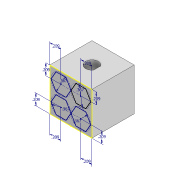
# Autodesk Inventor part: 615456 bevel gear lock A
Saved by Autodesk Inventor 2020 (Build 240168000, 168)
## iProperties
Created: 2019-11-11
Part Number: 615456 bevel gear lock A
Material: Generic
Document SubType Name: Modeling
Designer: ball
Density: 1 g/cm^3
Appearance: Default
Author: ball
Autodesk Inventor part; units mm, degrees
ref_plane "YZ Plane" through (0, 0, 0) normal (1, 0, 0) x (0, 1, 0)
ref_plane "XZ Plane" through (0, 0, 0) normal (0, 1, 0) x (-1, 0, 0)
ref_plane "XY Plane" through (0, 0, 0) normal (0, 0, 1) x (1, 0, 0)
sketch "Sketch1" plane through (0, 0, 0) normal (0, 1, 0) x (-1, 0, 0)
  line L0 (10, 0) -> (10, -10)
  line L1 (10, -10) -> (0, -10)
  line L2 (10, 0) -> (10, 10)
  line L3 (10, 10) -> (0, 10)
  line L4 (-10, 0) -> (-10, -10)
  line L5 (-10, -10) -> (0, -10)
  line L6 (-10, 0) -> (-10, 10)
  line L7 (-10, 10) -> (0, 10)
  arc A0 (-2.489, -1.6837) -> (-2.489, 1.6837) centre (0, 0) ccw
  line L8 (-2.489, -1.6837) -> (-2.489, 1.6837)
  dimension "d8" = 10
  dimension "d9" = 20
  dimension "d10" = 10
  dimension "d11" = 20
  dimension "d12" = 6.01
  dimension "d13" = 2.489
  constraints: 18 end point, 2 point on circle, 1 centre point, 1 coincident, 1 vertical
  measures "d8" distance from line of L1 point (0, 0)
  measures "d9" distance between parallel lines of L3 L1
  measures "d10" distance from line of L0 point (0, 0)
  measures "d11" distance between parallel lines of L4 L0
  measures "d12" diameter of A0
  measures "d13" distance from line of L8 point (0, 0)
extrude "Extrusion1" add sketch "Sketch1" along normal blind 20
sketch "Sketch2" plane through (-10, 0, 10) normal (0, 0, 1) x (1, 0, 0)
  circle A0 centre (5.2959, 14.7041) radius 4.6609 construction
  circle A1 centre (5.2959, 5.2959) radius 4.6609 construction
  circle A2 centre (14.7041, 14.7041) radius 4.6609 construction
  circle A3 centre (14.7041, 5.2959) radius 4.6609 construction
  line L0 (0, 0) -> (0, 20) projected
  line L1 (20, 0) -> (20, 20) projected
  line L2 (0, 20) -> (20, 20) projected
  line L3 (0, 0) -> (20, 0) projected
  line L4 (5.2959, 14.7041) -> (14.7041, 14.7041) construction
  line L5 (5.2959, 5.2959) -> (14.7041, 5.2959) construction
  line L6 (10, 14.7041) -> (7.648, 10.6302)
  line L7 (7.648, 10.6302) -> (2.9439, 10.6302)
  line L8 (2.9439, 10.6302) -> (0.5918, 14.7041)
  line L9 (0.5918, 14.7041) -> (2.9438, 18.778)
  line L10 (2.9438, 18.778) -> (7.6479, 18.778)
  line L11 (7.6479, 18.778) -> (10, 14.7041)
  line L12 (19.365, 14.7041) -> (17.0346, 10.6676)
  line L13 (17.0346, 10.6676) -> (12.3737, 10.6676)
  line L14 (12.3737, 10.6676) -> (10.0432, 14.7041)
  line L15 (10.0432, 14.7041) -> (12.3736, 18.7406)
  line L16 (12.3736, 18.7406) -> (17.0345, 18.7406)
  line L17 (17.0345, 18.7406) -> (19.365, 14.7041)
  line L18 (10, 5.2959) -> (7.648, 1.222)
  line L19 (7.648, 1.222) -> (2.9439, 1.222)
  line L20 (2.9439, 1.222) -> (0.5918, 5.2959)
  line L21 (0.5918, 5.2959) -> (2.9438, 9.3698)
  line L22 (2.9438, 9.3698) -> (7.6479, 9.3698)
  line L23 (7.6479, 9.3698) -> (10, 5.2959)
  line L24 (19.365, 5.2959) -> (17.0346, 1.2594)
  line L25 (17.0346, 1.2594) -> (12.3737, 1.2594)
  line L26 (12.3737, 1.2594) -> (10.0432, 5.2959)
  line L27 (10.0432, 5.2959) -> (12.3736, 9.3324)
  line L28 (12.3736, 9.3324) -> (17.0345, 9.3324)
  line L29 (17.0345, 9.3324) -> (19.365, 5.2959)
  point P0 (10, 0)
  dimension "d18" = 9.3218
  dimension "d19" = 9.3218
  dimension "d16" = 9.3218
  dimension "d17" = 9.3218
  dimension "d20" = 5.2959
  dimension "d21" = 5.2959
  dimension "d22" = 5.2959
  dimension "d23" = 5.2959
  dimension "d24" = 5.2959
  dimension "d25" = 5.2959
  dimension "d26" = 5.2959
  dimension "d27" = 5.2959
  constraints: 52 end point, 4 coincident, 2 centre point, 2 horizontal alignment, 2 midpoint, 1 point on line, 56 other
  measures "d16" diameter of A0
  measures "d17" diameter of A1
  measures "d20" distance from line of L4.start L0
  measures "d21" distance from line of L1 L4.end
  measures "d22" distance from line of L2 L4.start
  measures "d23" distance from line of L2 L4.end
  measures "d24" distance from line of L3 L5.start
  measures "d25" distance from line of L3 L5.end
  measures "d26" distance from line of L0 L5.start
  measures "d27" distance from line of L1 L5.end
body "Solid1"
